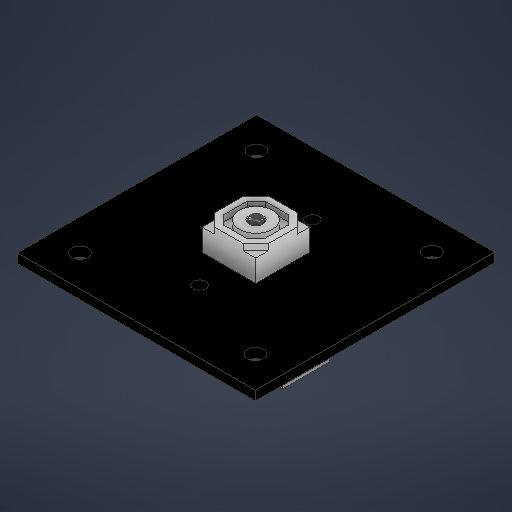
# Autodesk Inventor part: Camera
Saved by Autodesk Inventor 2025.1 (Build 291241000, 241)
## iProperties
Created: 2024-11-08
Part Number: Camera
Material: Generic
Document SubType Name: Modeling
Designer: jerem
Density: 1 g/cm^3
Appearance: Default
Author: jerem
Autodesk Inventor part; units mm, degrees
ref_plane "YZ Plane" through (0, 0, 0) normal (1, 0, 0) x (0, 1, 0)
ref_plane "XZ Plane" through (0, 0, 0) normal (0, 1, 0) x (-1, 0, 0)
ref_plane "XY Plane" through (0, 0, 0) normal (0, 0, 1) x (1, 0, 0)
sketch "Sketch1" plane through (0, 0, 0) normal (0, 1, 0) x (-1, 0, 0)
  line L0 (-19, -19.1) -> (19, -19.1)
  line L1 (19, -19.1) -> (19, 19.1)
  line L2 (19, 19.1) -> (-19, 19.1)
  line L3 (-19, 19.1) -> (-19, -19.1)
  line L4 (-19, -19.1) -> (19, 19.1) construction
  line L5 (19, -19.1) -> (-19, 19.1) construction
  line L6 (4.275, -4.2975) -> (-4.275, -4.2975)
  line L7 (-4.275, -4.2975) -> (-4.275, 4.2975)
  line L8 (-4.275, 4.2975) -> (4.275, 4.2975)
  line L9 (4.275, 4.2975) -> (4.275, -4.2975)
  line L10 (4.275, -4.2975) -> (-4.275, 4.2975) construction
  line L11 (-4.275, -4.2975) -> (4.275, 4.2975) construction
  circle A0 centre (14, 14.0737) radius 1.3
  circle A1 centre (0, 9) radius 1
  circle A2 centre (-14, 14.0737) radius 1.3
  circle A3 centre (0, -9) radius 1
  line L12 (0, 0) -> (0, 9) construction
  line L13 (0, -9) -> (0, 0) construction
  circle A4 centre (14, -14.0737) radius 1.3
  circle A5 centre (-14, -14.0737) radius 1.3
  line L14 (14, 14.0737) -> (14, -14.0737) construction
  line L15 (14, 14.0737) -> (-14, 14.0737) construction
  line L16 (-14, 14.0737) -> (-14, -14.0737) construction
  line L17 (4.275, -2.2975) -> (2.275, -4.2975)
  line L18 (-2.275, -4.2975) -> (-4.275, -2.2975)
  line L19 (-4.275, 2.2975) -> (-2.275, 4.2975)
  line L20 (2.275, 4.2975) -> (4.275, 2.2975)
  circle A6 centre (0, 0) radius 2.65
  circle A7 centre (0, 0) radius 1.15
  line L21 (1.8608, 3.2975) -> (-1.8608, 3.2975)
  line L22 (-1.8608, -3.2975) -> (1.8608, -3.2975)
  line L23 (1.8608, 3.2975) -> (3.275, 1.8833)
  line L24 (3.275, -1.8833) -> (1.8608, -3.2975)
  line L25 (-1.8608, -3.2975) -> (-3.275, -1.8833)
  line L26 (-3.275, 1.8833) -> (-1.8608, 3.2975)
  line L27 (3.775, 3.7949) -> (3.775, 3.7975)
  line L28 (3.775, -3.7975) -> (3.775, -3.7949)
  line L29 (3.275, -1.8833) -> (3.275, 1.8833)
  line L30 (-3.775, -3.7949) -> (-3.775, -3.7975)
  line L31 (-3.775, 3.7975) -> (-3.775, 3.7949)
  line L32 (-3.275, 1.8833) -> (-3.275, -1.8833)
  circle A8 centre (0, 0) radius 1
  dimension "d0" = 38
  dimension "d1" = 38.2
  dimension "d2" = 8.55
  dimension "d3" = 2
  dimension "d4" = 2
  dimension "d5" = 9
  dimension "d6" = 9
  dimension "d7" = 2.6
  dimension "d8" = 2.6
  dimension "d9" = 2.6
  dimension "d10" = 2.6
  dimension "d11" = 28
  dimension "d24" = 45
  dimension "d25" = 2
  dimension "d26" = 5.3
  dimension "d27" = 2.3
  dimension "d30" = 1
  dimension "d31" = 1
  dimension "d32" = 1
  dimension "d33" = 1
  dimension "d34" = 1
  dimension "d35" = 1
  dimension "d36" = 1
  dimension "d37" = 1
  dimension "d40" = 2
  constraints: 67 end point, 18 parallel, 17 point on line, 11 perpendicular, 9 centre point, 4 midpoint, 4 vertical, 3 coincident, 3 horizontal
  measures "d0" distance of L2.end L1.end
  measures "d1" distance of L0.end L1.end
  measures "d2" distance of L7.end L8.end
  measures "d3" diameter of A1
  measures "d4" diameter of A3
  measures "d5" distance of L12.start L13.start
  measures "d6" distance of L12.start L12.end
  measures "d7" diameter of A0
  measures "d8" diameter of A4
  measures "d9" diameter of A2
  measures "d10" diameter of A5
  measures "d11" distance of L14.start L15.end
  measures "d24" angle of L6 L17
  measures "d25" distance of L6.start L17.start
  measures "d26" diameter of A6
  measures "d27" diameter of A7
  measures "d30" distance between parallel lines of L8 L21
  measures "d31" distance between parallel lines of L20 L23
  measures "d32" distance between parallel lines of L17 L24
  measures "d33" distance between parallel lines of L18 L25
  measures "d34" distance between parallel lines of L19 L26
  measures "d35" distance between parallel lines of L9 L29
  measures "d36" distance between parallel lines of L6 L22
  measures "d37" distance between parallel lines of L7 L32
  measures "d40" diameter of A8
extrude "Extrusion1" add sketch "Sketch1" along normal blind 1.5 contours L3 L2 L1 L0 | L6 L17 L9 | L6 L18 L7 L19 L8 L20 L9 L17 | L6 L7 L18 | L20 L8 L9 | L7 L8 L19 | A6 | A7 | L23 L29 L24 L22 L25 L32 L26 L21 | A8
extrude "Extrusion2" add sketch "Sketch1" along normal blind 4.5 from surface at 1.5 contours L6 L17 L9 | L6 L18 L7 L19 L8 L20 L9 L17 | L6 L7 L18 | L20 L8 L9 | L7 L8 L19 | A6 | A7 | L23 L29 L24 L22 L25 L32 L26 L21 | A8
sketch "Sketch2" plane through (0, 0, 0) normal (0, -1, 0) x (1, 0, 0)
  line L0 (15, 10.78) -> (11.5, 10.78)
  line L1 (11.5, 10.78) -> (11.5, 3.28)
  line L2 (11.5, 3.28) -> (15, 3.28)
  line L3 (15, 3.28) -> (15, 10.78)
  line L4 (-19, 19.1) -> (19, 19.1) projected
  line L5 (19, 19.1) -> (19, -19.1) projected
  line L6 (11.9, 3.68) -> (11.9, 10.38)
  line L7 (11.9, 10.38) -> (14.6, 10.38)
  line L8 (14.6, 10.38) -> (14.6, 3.68)
  line L9 (14.6, 3.68) -> (11.9, 3.68)
  point P0 (0, 0)
  dimension "d16" = 8.32
  dimension "d17" = 7.5
  dimension "d18" = 3.5
  dimension "d19" = 4
  dimension "d23" = 0.4
  constraints: 16 end point, 4 parallel, 2 perpendicular, 1 horizontal, 3 other
  measures "d16" distance between parallel lines of L4 L0
  measures "d17" distance of L0.end L1.end
  measures "d18" distance of L1.end L2.end
  measures "d19" distance between parallel lines of L5 L3
  measures "d23" distance between parallel lines of L1 L6
extrude "Extrusion3" add sketch "Sketch2" along normal blind 4.5
extrude "Extrusion4" cut sketch "Sketch1" against normal blind 1 from surface at 6 contours L6 L17 L9 | L6 L7 L18 | L20 L8 L9 | L7 L8 L19 | L23 L29 L24 L22 L25 L32 L26 L21
extrude "Extrusion5" cut sketch "Sketch1" against normal blind 1 from surface at 6 contours A7 | A8
extrude "Extrusion6" add sketch "Sketch1" along normal blind 1.5 from surface at 5 contours A8
fillet "Fillet1" radius 0.5 1 edges at (1, 6.5, 0) curvature continuous yes
equation "\"d4\" = d3"
equation "\"d5\" = d6"
equation "\"d8\" = d7"
equation "\"d9\" = d7"
equation "\"d10\" = d7"
equation "\"d30\" = d35"
equation "\"d31\" = d35"
equation "\"d32\" = d35"
equation "\"d33\" = d35"
equation "\"d34\" = d35"
equation "\"d36\" = d35"
equation "\"d37\" = d36"
body "Solid1"
